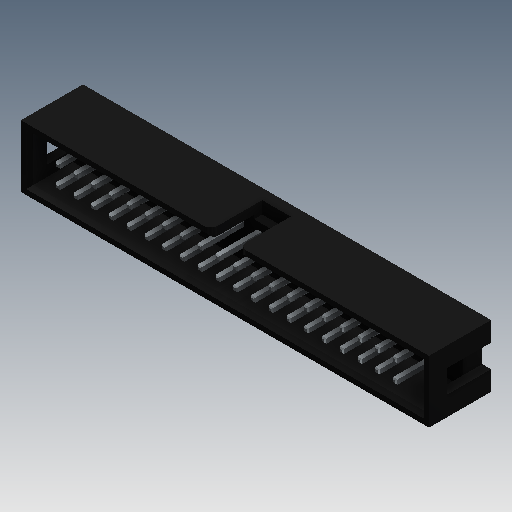
# Autodesk Inventor part: ide male connector
Saved by Autodesk Inventor 2019.1 (Build 231200000, 200)
## iProperties
Company: Autodesk Asia Pte. Ltd.
Created: 2005-12-05
Part Number: ide male connector
Document SubType Name: Modeling
Designer: Simon.Ng@autodesk.com
Density: 1 g/cm^3
Material: Generic
Mass: 2.38693 g
Surface Area: 35.2874 cm^2
Volume: 2.38693 cm^3
Appearance: Glossy - Black
Title: PC Demo
Author: Simon.Ng@autodesk.com
Autodesk Inventor part; units mm, degrees
ref_plane "YZ Plane" through (0, 0, 0) normal (1, 0, 0) x (0, 1, 0)
ref_plane "XZ Plane" through (0, 0, 0) normal (0, 1, 0) x (-1, 0, 0)
ref_plane "XY Plane" through (0, 0, 0) normal (0, 0, 1) x (1, 0, 0)
sketch "Sketch1" plane through (0, 0, 0) normal (0, 0, 1) x (1, 0, 0)
  line L0 (0, 7.112) -> (0, -5.334) projected
  line L1 (-35.052, 0) -> (46.736, 0) projected
  line L2 (-29.21, 4.445) -> (29.21, 4.445)
  line L3 (29.21, 4.445) -> (29.21, -4.445)
  line L4 (29.21, -4.445) -> (-29.21, -4.445)
  line L5 (-29.21, -4.445) -> (-29.21, 4.445)
  dimension "d0" = 58.42
  dimension "d1" = 8.89
  constraints: 8 end point, 2 parallel, 1 horizontal, 1 perpendicular, 2 other
  measures "d0" distance of L2.start L2.end
  measures "d1" distance of L4.end L2.start
extrude "Extrusion1" add sketch "Sketch1" along normal blind 8.89
shell "Shell1" thickness 0.4 removed faces 1 at (-9.7367, 1.4817, 8.89) ; own thickness 2.69 on faces at (-9.7367, 1.4817, 0) ; own thickness 1.27 on faces at (29.21, 1.4817, 5.9267) (-29.21, -1.4817, 2.9633) ; own thickness 1.245 on faces at (9.7367, -4.445, 2.9633) (-9.7367, 4.445, 2.9633)
sketch "Sketch2" plane through (29.21, -4.445, 0) normal (1, 0, 0) x (0, 0, -1)
  line L0 (0, 8.89) -> (0, 0) projected
  line L1 (-11.557, 4.445) -> (0.889, 4.445) projected
  line L2 (-2.69, 7.645) -> (-2.69, 1.245) projected
  line L3 (0, 6.096) -> (-6.35, 6.096)
  line L4 (-6.35, 6.096) -> (-6.35, 2.794)
  line L5 (-6.35, 2.794) -> (0, 2.794)
  line L6 (0, 2.794) -> (0, 6.096)
  dimension "d6" = 6.35
  dimension "d7" = 3.302
  constraints: 8 end point, 2 parallel, 1 horizontal, 1 perpendicular, 1 point on line, 1 other
  measures "d6" distance of L3.start L3.end
  measures "d7" distance of L3.end L4.end
extrude "Extrusion2" cut sketch "Sketch2" against normal up to surface (1.27 mm away)
sketch "Sketch3" plane through (-29.21, 4.445, 0) normal (0, 1, 0) x (1, 0, 0)
  line L0 (0, -8.89) -> (58.42, -8.89) projected
  line L1 (29.21, 0.889) -> (29.21, -11.557) projected
  line L2 (27.178, -8.89) -> (31.242, -8.89)
  line L3 (31.242, -8.89) -> (31.242, -1.524)
  line L4 (27.178, -1.524) -> (27.178, -8.89)
  line L5 (31.242, -1.524) -> (27.178, -1.524)
  dimension "d10" = 4.064
  dimension "d31" = 7.366
  constraints: 8 end point, 2 perpendicular, 1 horizontal, 1 parallel, 1 point on line, 1 other
  measures "d10" distance of L2.start L2.end
  measures "d31" distance of L2.end L3.end
extrude "Extrusion3" cut sketch "Sketch3" against normal blind 1.778
sketch "Sketch4" plane through (-27.94, 3.2, 2.69) normal (0, 0, 1) x (1, 0, 0)
  line L0 (51.755, -1.57) -> (52.385, -1.57)
  line L1 (52.385, -1.57) -> (52.385, -2.2)
  line L2 (52.385, -2.2) -> (51.755, -2.2)
  line L3 (51.755, -2.2) -> (51.755, -1.57)
  line L4 (51.755, -4.2) -> (52.385, -4.2)
  line L5 (52.385, -4.2) -> (52.385, -4.83)
  line L6 (52.385, -4.83) -> (51.755, -4.83)
  line L7 (51.755, -4.83) -> (51.755, -4.2)
  line L8 (29.972, -0.533) -> (25.908, -0.533) projected
  line L9 (55.88, -6.4) -> (0, -6.4) projected
  line L10 (27.94, -6.4) -> (27.94, -0.533)
  line L11 (52.07, -2.2) -> (52.07, -4.2) construction
  dimension "d18" = 0.63
  dimension "d32" = 48.26
  constraints: 20 end point, 4 midpoint, 4 parallel, 3 perpendicular, 2 collinear, 2 horizontal
  measures "d18" distance of L0.start L0.end
  measures "d32" diameter of L11 L10
extrude "Extrusion4" add sketch "Sketch4" along normal blind 6.1
chamfer "Chamfer1" distance 0.15 angle 45 8 edges at (24.13, 1, 8.79) (23.815, 1.315, 8.79) (24.13, 1.63, 8.79) (24.445, 1.315, 8.79) (24.445, -1.315, 8.79) (24.13, -1, 8.79) (23.815, -1.315, 8.79) (24.13, -1.63, 8.79)
pattern_linear "Rectangular Pattern2" count 20 spacing 2.54 along (-1, 0, 0) of "Extrusion4", "Chamfer1"
sketch "Sketch5" plane through (-29.21, -4.445, 0) normal (-1, 0, 0) x (0, 0, 1)
  line L0 (0, 0) -> (0, 8.89) projected
  line L1 (0, 6.096) -> (6.35, 6.096)
  line L2 (6.35, 6.096) -> (6.35, 2.794)
  line L3 (6.35, 2.794) -> (0, 2.794)
  line L4 (0, 2.794) -> (0, 6.096)
  point P0 (0, 4.445)
  point P1 (0, 4.445)
  dimension "d36" = 3.302
  dimension "d37" = 6.35
  constraints: 8 end point, 2 midpoint, 2 parallel, 1 coincident, 1 horizontal, 1 perpendicular, 1 point on line
  measures "d36" distance of L1.end L2.end
  measures "d37" distance of L2.end L3.end
extrude "Extrusion5" cut sketch "Sketch5" against normal up to surface (1.27 mm away)
chamfer "Chamfer2" distance 0.5 angle 45 5 edges at (0, -3.2, 8.89) (27.94, 0, 8.89) (14.986, 3.2, 8.89) (-14.986, 3.2, 8.89) (-27.94, 0, 8.89)
fillet "Fillet1" radius 1 2 edges at (2.032, 4.0725, 8.89) (-2.032, 4.0725, 8.89)
body "Solid1"
